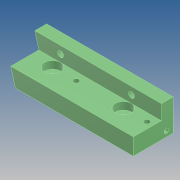
# Autodesk Inventor part: KB33-046-003-003 - Накладка на рычаг
Saved by Autodesk Inventor 2020 (Build 240168000, 168)
## iProperties
Created: 2021-06-25
Part Number: KB33-046-003-003 - Накладка на рычаг
Material: Пластик АБС
Document SubType Name: Modeling
Designer: Петров Иван
Mass: 31.64 g
Surface Area: 97.0231 cm^2
Volume: 29.8491 cm^3
Density: 1.06 g/cm^3
Appearance: Гладкий — темный травянисто-зеленый
Author: Петров Иван
Autodesk Inventor part; units mm, degrees
ref_plane "YZ Plane" through (0, 0, 0) normal (1, 0, 0) x (0, 1, 0)
ref_plane "XZ Plane" through (0, 0, 0) normal (0, 1, 0) x (-1, 0, 0)
ref_plane "XY Plane" through (0, 0, 0) normal (0, 0, 1) x (1, 0, 0)
sketch "Эскиз1" plane through (0, 0, 0) normal (0, 1, 0) x (-1, 0, 0)
  line L0 (-40, 13.5) -> (40, 13.5)
  line L1 (40, 13.5) -> (40, -13.5)
  line L2 (40, -13.5) -> (-40, -13.5)
  line L3 (-40, -13.5) -> (-40, 13.5)
  line L4 (-40, 13.5) -> (40, -13.5) construction
  line L5 (40, 13.5) -> (-40, -13.5) construction
  point P0 (0, 0)
  dimension "d0" = 80
  dimension "d1" = 27
  constraints: 12 end point, 2 midpoint, 2 parallel, 1 horizontal, 1 perpendicular
  measures "d0" distance of L1.end L2.end
  measures "d1" distance of L0.end L1.end
extrude "Выдавливание1" add sketch "Эскиз1" along normal blind 11.29
draft "НаклГрань1" angle -15 pull direction (0, 1, 0) faces at (-40, 7.526667, -4.5) fixed edges at (-40, 0, 0)
sketch "Эскиз3" plane through (0, 11.29, 0) normal (0, 1, 0) x (1, 0, 0)
  line L0 (40, 13.5) -> (-43.025146, 13.5)
  line L1 (40, -13.5) -> (40, 13.5)
  line L2 (-43.025146, 13.5) -> (40, 13.5)
  line L3 (40, 13.5) -> (40, 5.5)
  line L4 (40, 5.5) -> (-43.025146, 5.5)
  line L5 (-43.025146, 5.5) -> (-43.025146, 13.5)
  point P0 (0, 0)
  dimension "d8" = 8
  constraints: 8 end point, 2 parallel, 1 horizontal, 1 perpendicular, 1 point on line
  measures "d8" distance of L2.end L3.end
extrude "Выдавливание3" add sketch "Эскиз3" along normal blind 10
draft "НаклГрань2" angle -15 pull direction (0, 1, 0) faces at (-43.025146, 14.623333, -10.833333) fixed edges at (-43.025146, 11.29, -9.5)
sketch "Эскиз4" plane through (0, 11.29, 0) normal (0, 1, 0) x (1, 0, 0)
  circle A0 centre (19.722768, 0) radius 1.85
  circle A1 centre (-12.277232, 0) radius 1.85
  circle A2 centre (-28.277232, 0) radius 1.85
  circle A3 centre (3.722768, 0) radius 1.85
  circle A4 centre (35.722768, 0) radius 1.85
  point P0 (0, 0)
extrude "Выдавливание4" cut sketch "Эскиз4" against normal blind 30.75 contours A0 | A1 | A2 | A4
sketch "Эскиз5" plane through (0, 11.29, 0) normal (0, 1, 0) x (1, 0, 0)
  circle A0 centre (-28.277232, 0) radius 1.85
  circle A1 centre (-28.277232, 0) radius 5.5
  line L0 (40, 5.5) -> (-43.025146, 5.5)
  circle A2 centre (19.722768, 0) radius 1.85
  circle A3 centre (19.722768, 0) radius 5.5
  point P0 (0, 0)
  constraints: 2 centre point, 2 coincident, 2 tangent
extrude "Выдавливание5" cut sketch "Эскиз5" against normal blind 5 contours A1 | A2 | A3
sketch "Эскиз6" plane through (40, 0, -13.5) normal (0, 0, -1) x (-1, 0, 0)
  line L0 (22.127232, 6.29) -> (18.427232, 6.29)
  line L1 (70.127232, 6.29) -> (66.427232, 6.29)
  line L2 (20.277232, 11.29) -> (68.277232, 11.29)
  line L3 (14.777232, 6.29) -> (25.777232, 6.29)
  line L4 (20.277232, 6.29) -> (20.277232, 16.29) construction
  circle A0 centre (20.277232, 16.29) radius 2
  line L5 (68.277232, 6.29) -> (68.277232, 16.29) construction
  circle A1 centre (68.277232, 16.29) radius 2
  point P0 (40, 0)
  dimension "d16" = 5
  dimension "d17" = 4
  dimension "d18" = 4
  constraints: 4 end point, 2 centre point, 2 coincident, 2 midpoint, 2 vertical
  measures "d16" distance from line of L2 L4.end
  measures "d17" diameter of A0
  measures "d18" diameter of A1
extrude "Выдавливание6" cut sketch "Эскиз6" against normal blind 30.75
ref_plane "РабПлоскость1" through (35, 0, 13.5) normal (1, 0, 0) x (0, 0, -1)
sketch "Эскиз7" plane through (35, 0, 13.5) normal (1, 0, 0) x (0, 0, -1)
  line L0 (27, 0) -> (0, 0)
  line L1 (22.395435, 0) -> (19.245435, 1.818653)
  line L2 (19.245435, 1.818653) -> (19.245435, 5.45596)
  line L3 (19.245435, 5.45596) -> (22.395435, 7.274613)
  line L4 (22.395435, 7.274613) -> (25.545435, 5.45596)
  line L5 (25.545435, 5.45596) -> (25.545435, 1.818653)
  line L6 (25.545435, 1.818653) -> (22.395435, 0)
  line L7 (27, 0) -> (27, 21.29)
  line L8 (25.545435, 1.818653) -> (25.545435, 0)
  line L9 (19.245435, 1.818653) -> (19.245435, 0)
  point P0 (13.5, 0)
  point P1 (22.395435, 3.637307)
  dimension "d22" = 6.3
  constraints: 16 end point, 3 point on line, 2 perpendicular, 1 parallel, 13 other
  measures "d22" distance between parallel lines of L2 L5
extrude "Выдавливание7" cut sketch "Эскиз7" along normal mid plane 5
sketch "Эскиз9" plane through (40, 0, 13.5) normal (1, 0, 0) x (0, 0, -1)
  line L0 (27, 0) -> (0, 0)
  line L1 (22.395435, 0) -> (19.245435, 1.818653)
  line L2 (19.245435, 1.818653) -> (19.245435, 5.45596)
  line L3 (19.245435, 5.45596) -> (22.395435, 7.274613)
  line L4 (22.395435, 7.274613) -> (25.545435, 5.45596)
  line L5 (25.545435, 5.45596) -> (25.545435, 1.818653)
  line L6 (25.545435, 1.818653) -> (22.395435, 0)
  line L7 (27, 0) -> (27, 21.29)
  line L8 (25.545435, 1.818653) -> (25.545435, 0)
  line L9 (19.245435, 1.818653) -> (19.245435, 0)
  circle A0 centre (22.395435, 3.637307) radius 1.5
  point P0 (13.5, 0)
  point P1 (13.5, 0)
  dimension "d27" = 6.3
  dimension "d28" = 3
  constraints: 20 end point, 3 point on line, 2 perpendicular, 1 centre point, 1 coincident, 1 parallel, 13 other
  measures "d27" distance between parallel lines of L2 L5
  measures "d28" diameter of A0
extrude "Выдавливание8" cut sketch "Эскиз9" against normal blind 5 contours A0
equation "\"d18\" = d17"
